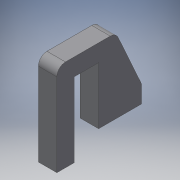
# Autodesk Inventor part: TrayPanelJ
Saved by Autodesk Inventor 2017 (Build 210142000, 142)
## iProperties
Created: 2019-06-26
Part Number: TrayPanelJ
Material: Generic
Document SubType Name: Modeling
Designer: DDeGo
Density: 1 g/cm^3
Appearance: Default
Author: DDeGo
Autodesk Inventor part; units mm, degrees
ref_plane "YZ Plane" through (0, 0, 0) normal (1, 0, 0) x (0, 1, 0)
ref_plane "XZ Plane" through (0, 0, 0) normal (0, 1, 0) x (-1, 0, 0)
ref_plane "XY Plane" through (0, 0, 0) normal (0, 0, 1) x (1, 0, 0)
sketch "Sketch1" plane through (0, 0, 0) normal (1, 0, 0) x (0, 1, 0)
  line L0 (0, 0) -> (0, 21.3)
  line L1 (0, 21.3) -> (13.7, 21.3)
  line L2 (19.7, 4) -> (9.7, 4)
  line L3 (9.7, 4) -> (9.7, 17.3)
  line L4 (9.7, 17.3) -> (4, 17.3)
  line L5 (4, 17.3) -> (4, 0)
  line L6 (4, 0) -> (0, 0)
  line L7 (13.7, 21.3) -> (19.7, 8)
  line L8 (19.7, 8) -> (19.7, 4)
  dimension "d0" = 4
  dimension "d1" = 4
  dimension "d2" = 5.7
  dimension "d4" = 4
  dimension "d5" = 10
  dimension "d6" = 13.3
  dimension "d9" = 4
  dimension "d11" = 4
  constraints: 18 end point, 5 perpendicular, 2 vertical, 1 parallel
  measures "d0" distance between parallel lines of L1 L4
  measures "d1" distance between parallel lines of L0 L5
  measures "d2" distance between parallel lines of L3 L5
  measures "d4" distance from line of L1.end L3
  measures "d5" distance of L2.start L2.end
  measures "d6" distance between parallel lines of L4 L2
  measures "d9" distance of L7.end L2.start
  measures "d11" distance between parallel lines of L6 L2
extrude "Extrusion1" add sketch "Sketch1" along normal blind 4.3
fillet "Fillet1" radius 2 3 edges at (2.15, 0, 21.3) (2.15, 13.7, 21.3) (2.15, 19.7, 8)
body "Solid1"
